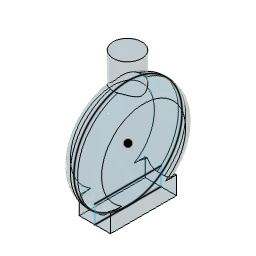
Electromagnet Holder One 100lb v5 (Autodesk Fusion 360 archive; units mm, degrees)
design "Ferrofluid Bottle"
Autodesk Fusion 360 part; units mm, degrees
sketch "Sketch1" plane through (0, 0, 0) normal (1, 0, 0) x (0, 1, 0)
  circle A0 centre (0, 0) radius 45
  line L0 (27.4205, -45) -> (-27.5795, -45)
  line L1 (-27.5795, -45) -> (-27.5795, -30)
  line L2 (-27.5795, -30) -> (27.4205, -30)
  line L3 (27.4205, -30) -> (27.4205, -45)
  dimension "d8" = 90
  dimension "d10" = 55
  dimension "d11" = 15
  constraint coincident A0.centre origin
  constraint horizontal L0
  constraint vertical L1
  constraint horizontal L2
  constraint vertical L3
  constraint tangent A0 L0
  measures "d8" diameter of A0
  measures "d10" distance of L0.start L0.end
  measures "d11" distance of L0.start L2.end
cylinder "CylinderPrimitive1" add diameter 90 height 13 placed x (0, 0, -1) y (0, 1, 0) z (1, 0, 0) at (0, 0, 0) makes body 1
fillet "Fillet1" radius 10 1 edges at (13, -16.2727, 41.9547) on bodies 1
extrude "Extrude1" add sketch "Sketch1" along normal blind 13 contours A0 L1 L2 L3 | A0 L0 L1 | A0 L0 L3 picked at (-0.053, -35) bodies 1
cylinder "CylinderPrimitive2" add diameter 90 height 13 placed x (0, 0, 1) y (0, 1, 0) z (-1, 0, 0) at (0, 0, 0) bodies 1
fillet "Fillet2" radius 10 1 edges at (-13, -16.2727, -41.9547) on bodies 1
extrude "Extrude2" add sketch "Sketch1" against normal blind 13 contours A0 L1 L2 L3 | A0 L0 L1 | A0 L0 L3 picked at (-0.053, -35) bodies 1
ref_plane "WorkPlane1" through (-0.4102, 0, 45) normal (0, 0, 1) x (0, 1, 0)
sketch "Sketch5" plane through (-0.4102, 0, 45) normal (0, 0, 1) x (1, 0, 0)
  circle A0 centre (0, 0) radius 12
  dimension "d26" = 24
  constraint coincident A0.centre origin
  measures "d26" diameter of A0
extrude "Extrude3" add sketch "Sketch5" against normal blind 10 bodies 1
extrude "Extrude4" add 1 faces at (0.1622, -3.9888, 45) along direction (0, 0, 1) blind 22 on bodies 1 bodies 1
copy_body "Body->Comp1" bodies 1 removing the originals makes body 2 in component "Component"
component "Component" placed x (1, 0, 0) y (0, 1, 0) z (0, 0, 1) at (0, 0, 0)
equation "start_dia = 80 mm" comment "Inner diameter"
equation "diameter = 90 mm" comment "Diameter of glass"
equation "base_length = 55 mm" comment "Length of base"
equation "base_depth = 26 mm" comment "Depth of base"
equation "top_dia = 24 mm" comment "Diameter of top opening"
equation "top_length = 22 mm" comment "Length of top"
equation "base_height = 15 mm" comment "Height of the tallest part of the base"
equation "d8 = diameter"
equation "d10 = base_length"
equation "d11 = base_height"
equation "d12 = base_depth / 2"
equation "d16 = diameter - start_dia"
equation "d17 = base_depth / 2"
equation "d19 = base_depth / 2"
equation "d23 = -base_depth / 2"
equation "d26 = top_dia"
equation "d29 = top_length"
